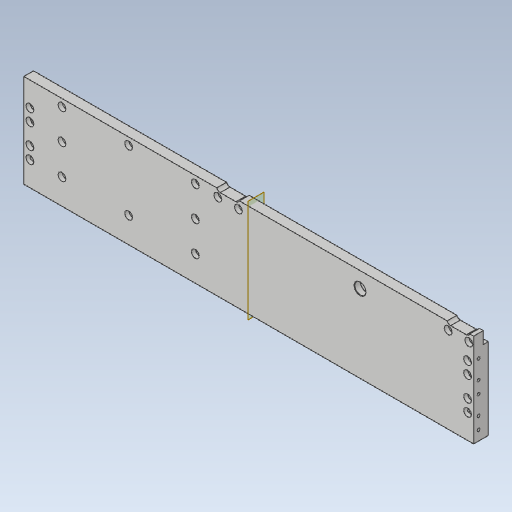
# Autodesk Inventor part: Frame Front
Saved by Autodesk Inventor 2020 (Build 240168000, 168)
## iProperties
Created: 2019-02-26
Part Number: Frame Front
Material: Generic
Document SubType Name: Modeling
Designer: LillaHunden
Density: 1 g/cm^3
Appearance: Default
Author: LillaHunden
Autodesk Inventor part; units mm, degrees
ref_plane "YZ Plane" through (0, 0, 0) normal (1, 0, 0) x (0, 1, 0)
ref_plane "XZ Plane" through (0, 0, 0) normal (0, 1, 0) x (-1, 0, 0)
ref_plane "XY Plane" through (0, 0, 0) normal (0, 0, 1) x (1, 0, 0)
sketch "Sketch1" plane through (0, 0, 0) normal (0, 0, 1) x (1, 0, 0)
  line L0 (211.8284, 9.9823) -> (215, 9.9823) projected
  line L1 (215, 9.9823) -> (215, -67) projected
  line L2 (215, -67) -> (-156, -67) projected
  line L3 (-156, -67) -> (-156, 9.9823) projected
  arc A0 (193.1716, 9.9823) -> (196, 7.9823) centre (196, 10.9823) ccw projected
  line L4 (196, 7.9823) -> (209, 7.9823) projected
  arc A1 (209, 7.9823) -> (211.8284, 9.9823) centre (209, 10.9823) ccw projected
  arc A2 (3.1716, 9.9823) -> (6, 7.9823) centre (6, 10.9823) ccw projected
  line L5 (6, 7.9823) -> (19, 7.9823) projected
  arc A3 (19, 7.9823) -> (21.8284, 9.9823) centre (19, 10.9823) ccw projected
  arc A4 (46.83, -62.57) -> (52.03, -62.57) centre (49.43, -62.57) ccw projected
  line L6 (52.03, -62.57) -> (52.03, -46.57) projected
  arc A5 (52.03, -46.57) -> (46.83, -46.57) centre (49.43, -46.57) ccw projected
  line L7 (46.83, -46.57) -> (46.83, -62.57) projected
  arc A6 (46.83, -15.43) -> (52.03, -15.43) centre (49.43, -15.43) ccw projected
  line L8 (52.03, -15.43) -> (52.03, 0.57) projected
  arc A7 (52.03, 0.57) -> (46.83, 0.57) centre (49.43, 0.57) ccw projected
  line L9 (46.83, 0.57) -> (46.83, -15.43) projected
  arc A8 (93.97, -15.43) -> (99.17, -15.43) centre (96.57, -15.43) ccw projected
  line L10 (99.17, -15.43) -> (99.17, 0.57) projected
  arc A9 (99.17, 0.57) -> (93.97, 0.57) centre (96.57, 0.57) ccw projected
  line L11 (93.97, 0.57) -> (93.97, -15.43) projected
  arc A10 (93.97, -62.57) -> (99.17, -62.57) centre (96.57, -62.57) ccw projected
  line L12 (99.17, -62.57) -> (99.17, -46.57) projected
  arc A11 (99.17, -46.57) -> (93.97, -46.57) centre (96.57, -46.57) ccw projected
  line L13 (93.97, -46.57) -> (93.97, -62.57) projected
  circle A12 centre (21, 3.7521) radius 3.25 projected
  circle A13 centre (211, 3.7521) radius 3.25 projected
  circle A14 centre (194, 3.7521) radius 3.25 projected
  circle A15 centre (4, 3.7521) radius 3.25 projected
  circle A16 centre (-123.8333, -6.3333) radius 3.25 projected
  circle A17 centre (-123.8333, -14.3333) radius 3.25 projected
  circle A18 centre (26.1667, -14.3333) radius 3.25 projected
  circle A19 centre (-3.8333, -14.3333) radius 3.25 projected
  circle A20 centre (-33.8333, -6.3333) radius 3.25 projected
  circle A21 centre (-63.8333, -14.3333) radius 3.25 projected
  circle A22 centre (-93.8333, -14.3333) radius 3.25 projected
  circle A23 centre (-93.8333, -6.3333) radius 3.25 projected
  circle A24 centre (-63.8333, -6.3333) radius 3.25 projected
  circle A25 centre (-33.8333, -14.3333) radius 3.25 projected
  circle A26 centre (-3.8333, -6.3333) radius 3.25 projected
  circle A27 centre (26.1667, -6.3333) radius 3.25 projected
  arc A28 (81.6, -25.6) -> (64.4, -25.6) centre (73, -25.6) ccw projected
  line L14 (64.4, -25.6) -> (64.4, -36.4) projected
  arc A29 (64.4, -36.4) -> (81.6, -36.4) centre (73, -36.4) ccw projected
  line L15 (81.6, -36.4) -> (81.6, -25.6) projected
  circle A30 centre (121.3, -3.0177) radius 8.6 projected
  line L16 (21.8284, 9.9823) -> (193.1716, 9.9823) projected
  line L17 (-156, 9.9823) -> (3.1716, 9.9823) projected
  point P0 (0, 0)
  point P1 (196, 10.9823)
  point P2 (19, 10.9823)
  point P3 (196, 10.9823)
  point P4 (6, 10.9823)
  point P5 (19, 10.9823)
  point P6 (209, 10.9823)
  point P7 (196, 10.9823)
  point P8 (6, 10.9823)
  point P9 (19, 10.9823)
extrude "Extrusion1" add sketch "Sketch1" along normal blind 12 contours L0 L1 L2 L3 L17 A2 L5 A3 L16 A0 L4 A1 | L7 A5 L6 A4 | L9 A7 L8 A6 | L11 A9 L10 A8 | L13 A11 L12 A10 | A12 | A13 | A14 | A15 | A16 | A17 | A18 | A19 | A20 | A21 | A22 | A23 | A24 | A25 | A26 | A27 | L15 A29 L14 A28 | A30
sketch "Sketch2" plane through (215, -67, 0) normal (1, 0, 0) x (0, 0, -1)
  line L0 (280, 67) -> (-4, 67) construction
  line L1 (280, 67) -> (280, 76.9823) construction
  line L2 (-4, 76.9823) -> (280, 76.9823) construction
  line L3 (0, 0) -> (0, 76.9823) construction
  line L4 (0, 76.9823) -> (-12, 76.9823) construction
  line L5 (-12, 0) -> (-12, 76.9823) construction
  line L6 (0, 0) -> (-12, 0) construction
  line L7 (0, 76.9823) -> (0, 0) projected
  line L8 (0, 76.9823) -> (-2, 76.9823)
  line L9 (-2, 76.9823) -> (-2, 67) construction
  line L10 (-2, 67) -> (0, 67)
  line L11 (0, 67) -> (0, 76.9823)
  line L12 (-4, 76.9823) -> (-4, 67) projected
  line L13 (0, 76.9823) -> (-12, 76.9823) projected
  line L14 (0, 67) -> (-4, 67)
  line L15 (-4, 67) -> (-4, 76.9823)
  line L16 (-4, 76.9823) -> (0, 76.9823)
  line L17 (0, 76.9823) -> (0, 67)
  point P0 (0, 67)
  dimension "d48" = 4
  constraints: 16 end point, 4 parallel, 2 horizontal, 2 perpendicular, 1 point on line
  measures "d48" distance of L15.end L16.end
extrude "Extrusion2" cut sketch "Sketch2" against normal through all
sketch "Sketch3" plane through (0, 0, 0) normal (0, 0, -1) x (-1, 0, 0)
  point P0 (0, 0)
sketch "Sketch4" plane through (0, 0, 0) normal (0, 0, -1) x (-1, 0, 0)
  circle A0 centre (-121.3, -3.0177) radius 2.5 construction
  arc A1 (-127.7, -10.7014) -> (-114.9, -10.7014) centre (-121.3, -3.0177) ccw
  arc A2 (-127.7, -10.7014) -> (-157.269, 0) centre (-157.269, -46.2018) ccw
  line L0 (156, 0) -> (-215, 0) projected
  line L1 (-121.3, -3.0177) -> (-121.3, 6.9823) construction
  arc A3 (-85.331, 0) -> (-114.9, -10.7014) centre (-85.331, -46.2018) ccw
  line L2 (-157.269, 0) -> (-85.331, 0)
  line L3 (-215, 0) -> (156, 0) projected
  line L4 (-157.269, 0) -> (-215, 0)
  line L5 (-85.331, 0) -> (156, 0)
  line L6 (156, 9.9823) -> (156, -67) projected
  point P0 (0, 0)
  point P1 (-3.1716, 9.9823)
  point P2 (-21.8284, 9.9823)
  dimension "d4" = 20
  dimension "d59" = 46.2018
  dimension "d60" = 5
  dimension "d61" = 277.3
  dimension "d62" = 10.7014
  dimension "d63" = 6.9823
  constraints: 8 end point, 6 point on circle, 4 centre point, 3 symmetric about line, 3 tangent, 2 collinear, 1 coincident, 1 perpendicular, 1 point on line, 1 other
  measures "d4" diameter of A1
  measures "d59" radius of A3
  measures "d60" diameter of A0
  measures "d61" distance from line of L6.start L1
  measures "d62" distance from line of A1.end L0
  measures "d63" distance from line of L1.end L0
extrude "Extrusion3" cut sketch "Sketch4" against normal up to surface (4 mm away)
sketch "Sketch5" plane through (215, 0, 4) normal (0, 0, -1) x (-1, 0, 0)
  circle A0 centre (4825.1843, -5.0177) radius 4.7125
  circle A1 centre (93.7, -3.0177) radius 4.4625 projected
  point P0 (215, 0)
  constraints: 1 centre point
extrude "Extrusion4" cut sketch "Sketch5" against normal through all both and the other way through all
chamfer "Chamfer1" distance 0.5 angle 45 1 edges at (125.7625, -3.0177, 12)
sketch "Sketch6" plane through (0, 0, 12) normal (0, 0, 1) x (1, 0, 0)
  circle A0 centre (211, 3.7521) radius 1.7 projected
  circle A1 centre (194, 3.7521) radius 1.7 projected
  circle A2 centre (4, 3.7521) radius 1.7 projected
  circle A3 centre (21, 3.7521) radius 1.7 projected
  point P0 (0, 0)
hole "Hole1" at (211, 3.7521, 12) at (194, 3.7521, 12) at (21, 3.7521, 12) at (4, 3.7521, 12) direction (0, 0, -1) diameter 3.4 depth 14.2 counterbore diameter 6.5 counterbore depth 3.4 clearance for "Socket Head Cap Screw ISO 4762" size "M3" standard "ISO"
sketch "Sketch7" plane through (215, 0, 4) normal (0, 0, -1) x (-1, 0, 0)
  circle A0 centre (93.7, -3.0177) radius 4.6625
  circle A1 centre (93.7, -3.0177) radius 3.475 projected
  circle A2 centre (93.7, -3.0177) radius 4.7625 projected
  point P0 (215, 0)
  dimension "d23" = 0.1
  constraints: 1 centre point
  measures "d23" radial gap between concentric circles of A2 A0
extrude "Extrusion5" cut sketch "Sketch7" along normal mid plane 30 contours A0 | A1
sketch "Sketch8" plane through (0, 0, 12) normal (0, 0, 1) x (1, 0, 0)
  line L0 (-124.5561, 3.9823) -> (-14.5561, 3.9823) construction
  line L1 (-14.5561, 3.9823) -> (-14.5561, -46.0177) construction
  line L2 (-14.5561, -46.0177) -> (-124.5561, -46.0177) construction
  line L3 (-124.5561, -46.0177) -> (-124.5561, 3.9823) construction
  line L4 (3.1716, 9.9823) -> (-156, 9.9823) projected
  point P0 (0, 0)
  point P1 (-124.5561, -21.0177)
  point P2 (-69.5561, -46.0177)
  point P3 (-69.5561, 3.9823)
  point P4 (-14.5561, -21.0177)
  dimension "d26" = 110
  dimension "d27" = 50
  dimension "d28" = 6
  constraints: 8 end point, 4 coincident, 4 midpoint, 2 parallel, 1 horizontal, 1 perpendicular
  measures "d26" distance of L1.end L2.end
  measures "d27" distance of L0.end L1.end
  measures "d28" distance between parallel lines of L4 L0
hole "Hole2" at (-14.5561, -21.0177, 12) at (-69.5561, 3.9823, 12) at (-69.5561, -46.0177, 12) at (-124.5561, -21.0177, 12) at (-14.5561, 3.9823, 12) at (-14.5561, -46.0177, 12) at (-124.5561, -46.0177, 12) at (-124.5561, 3.9823, 12) direction (0, 0, -1) diameter 2.459 end through all counterbore diameter 6.5 counterbore depth 3.4 thread size "M3x0.5" class "6H" standard "ISO Metric profile"
sketch "Sketch9" plane through (0, 0, 12) normal (0, 0, 1) x (1, 0, 0)
  line L0 (-156, -67) -> (215, -67) projected
  line L1 (3.1716, 9.9823) -> (-156, 9.9823) projected
  line L2 (-156, 9.9823) -> (-156, -67) projected
  point P0 (0, 0)
  point P1 (-151, -10.0177)
  point P2 (-151, -20.0177)
  point P3 (-151, -37)
  point P4 (-151, -47)
  dimension "d36" = 20
  dimension "d37" = 10
  dimension "d38" = 20
  dimension "d39" = 10
  dimension "d40" = 5
  constraints: 3 vertical alignment
  measures "d36" distance from line of L0 point (-151, -47)
  measures "d37" distance of point (-151, -47) point (-151, -37)
  measures "d38" distance from line of L1 point (-151, -10.018)
  measures "d39" distance of point (-151, -10.018) point (-151, -20.018)
  measures "d40" distance from line of L2 point (-151, -10.018)
hole "Hole3" at (-151, -47, 12) at (-151, -37, 12) at (-151, -20.0177, 12) at (-151, -10.0177, 12) direction (0, 0, -1) diameter 2.459 end through all counterbore diameter 6.5 counterbore depth 3.4 thread size "M3x0.5" class "6H" standard "ISO Metric profile"
ref_plane "Work Plane1" through (29.5, -67, 12) normal (-1, 0, 0) x (0, 0, 1)
mirror "Mirror1" about plane through (29.5, -67, 12) normal (-1, 0, 0) of "Hole3"
sketch "Sketch10" plane through (215, 0, 4) normal (0, 0, -1) x (-1, 0, 0)
  circle A0 centre (93.7, -3.0177) radius 4.4625 construction
  circle A1 centre (93.7, -3.0177) radius 4.775
  point P0 (215, 0)
  point P1 (96.9875, 0)
  point P2 (90.4125, 0)
  dimension "d49" = 9.55
  constraints: 1 centre point, 1 coincident
  measures "d49" diameter of A1
extrude "Extrusion6" cut sketch "Sketch10" against normal blind 3
sketch "Sketch12" plane through (-156, -67, 12) normal (-1, 0, 0) x (0, 0, 1)
  point P0 (-4.05, 68.9823)
  point P1 (-295.95, 68.9823)
  point P2 (-295.95, 58.9823)
  point P3 (-295.95, 43.4912)
  point P4 (-295.95, 33.4912)
  point P5 (-295.95, 18)
  point P6 (-295.95, 8)
  point P7 (-4.05, 33.4912)
  point P8 (-4.05, 43.4912)
  point P9 (-4.05, 8)
  point P10 (-4.05, 18)
  point P11 (-4.05, 58.9823)
hole "Hole5" at (-156, 1.9823, 7.95) at (-156, 1.9823, -283.95) at (-156, -8.0177, -283.95) at (-156, -23.5088, -283.95) at (-156, -33.5088, -283.95) at (-156, -49, -283.95) at (-156, -59, -283.95) at (-156, -33.5088, 7.95) at (-156, -23.5088, 7.95) at (-156, -59, 7.95) at (-156, -49, 7.95) at (-156, -8.0177, 7.95) direction (1, 0, 0) diameter 2.459 depth 8 tip angle 120 thread size "M3x0.5" class "6H" standard "ISO Metric profile"
sketch "Sketch14" plane through (215, -67, 12) normal (1, 0, 0) x (0, 0, -1)
  point P0 (4.05, 8)
  point P1 (4.05, 18)
  point P2 (4.05, 33.4912)
  point P3 (4.05, 43.4912)
  point P4 (4.05, 58.9823)
hole "Hole8" at (215, -59, 7.95) at (215, -49, 7.95) at (215, -33.5088, 7.95) at (215, -23.5088, 7.95) at (215, -8.0177, 7.95) direction (-1, 0, 0) diameter 2.459 depth 8 tip angle 120 thread size "M3x0.5" class "6H" standard "ISO Metric profile"
equation "\"d38\" = d36"
equation "\"d39\" = d37"
body "Solid1"
